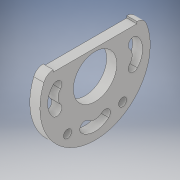
# Autodesk Inventor part: ballast_tengah
Saved by Autodesk Inventor 2019 (Build 230136000, 136)
## iProperties
Created: 2020-07-18
Part Number: ballast_tengah
Material: Generic
Document SubType Name: Modeling
Designer: Agus Prayudi
Density: 1 g/cm^3
Appearance: Default
Author: Agus Prayudi
Autodesk Inventor part; units mm, degrees
ref_plane "YZ Plane" through (0, 0, 0) normal (1, 0, 0) x (0, 1, 0)
ref_plane "XZ Plane" through (0, 0, 0) normal (0, 1, 0) x (-1, 0, 0)
ref_plane "XY Plane" through (0, 0, 0) normal (0, 0, 1) x (1, 0, 0)
sketch "Sketch1" plane through (0, 0, 0) normal (1, 0, 0) x (0, 1, 0)
  arc A0 (13.4228, -41.8269) -> (6.5772, -34.1731) centre (10, -38) ccw
  arc A1 (-13.4228, -41.8269) -> (13.4228, -41.8269) centre (0, -26.8197) ccw
  arc A2 (-6.5772, -34.1731) -> (-13.4228, -41.8269) centre (-10, -38) ccw
  arc A3 (-6.5772, -34.1731) -> (6.5772, -34.1731) centre (0, -26.8197) ccw
  arc A4 (-41.8269, -13.4228) -> (-34.1731, -6.5772) centre (-38, -10) ccw
  arc A5 (-41.8269, 13.4228) -> (-41.8269, -13.4228) centre (-26.8197, 0) ccw
  arc A6 (-34.1731, 6.5772) -> (-41.8269, 13.4228) centre (-38, 10) ccw
  arc A7 (-34.1731, 6.5772) -> (-34.1731, -6.5772) centre (-26.8197, 0) ccw
  arc A8 (-13.4228, 41.8269) -> (-6.5772, 34.1731) centre (-10, 38) ccw
  arc A9 (13.4228, 41.8269) -> (-13.4228, 41.8269) centre (0, 26.8197) ccw
  arc A10 (6.5772, 34.1731) -> (13.4228, 41.8269) centre (10, 38) ccw
  arc A11 (6.5772, 34.1731) -> (-6.5772, 34.1731) centre (0, 26.8197) ccw
  circle A12 centre (0, 0) radius 21.5
  circle A13 centre (-35.3988, 27.25) radius 3.5
  circle A14 centre (-35.3988, -27.25) radius 3.5
  arc A15 (20.2079, 50.6151) -> (20.2079, -50.6151) centre (0, 0) ccw
  line L0 (26.5, -41.328) -> (26.5, 41.328)
  arc A16 (26.5, 41.328) -> (20.2079, 50.6151) centre (16.5, 41.328) ccw
  arc A17 (20.2079, -50.6151) -> (26.5, -41.328) centre (16.5, -41.328) ccw
  point P0 (26.5, -47.6235)
  point P1 (26.5, 47.6235)
  dimension "d4" = 10
  dimension "d5" = 10
  constraints: 32 point on circle, 18 centre point, 4 tangent, 2 end point, 2 point on line
  measures "d4" radius of A16
  measures "d5" radius of A17
extrude "Extrusion1" add sketch "Sketch1" along normal blind 10
sketch "Sketch2" plane through (10, 0, 0) normal (1, 0, 0) x (0, 0, -1)
  line L0 (41.328, 26.5) -> (-41.328, 26.5) projected
  line L1 (0, 24.5) -> (41.328, 24.5)
  line L2 (41.328, 24.5) -> (41.328, 26.5)
  line L3 (0, 24.5) -> (-41.328, 24.5)
  line L4 (-41.328, 24.5) -> (-41.328, 26.5)
  point P0 (0, 0)
  constraints: 8 end point, 1 perpendicular
extrude "Extrusion2" cut sketch "Sketch2" against normal blind 10
sketch "Sketch3" plane through (10, 0, 0) normal (1, 0, 0) x (0, 0, -1)
  circle A0 centre (-27.25, -35.3988) radius 3.5 projected
  circle A1 centre (27.25, -35.3988) radius 3.5 projected
  circle A2 centre (-27.25, -35.3988) radius 4
  circle A3 centre (27.25, -35.3988) radius 4
  point P0 (0, 0)
  dimension "d11" = 8
  dimension "d12" = 8
  constraints: 2 centre point, 2 coincident
  measures "d11" diameter of A2
  measures "d12" diameter of A3
extrude "Extrusion3" cut sketch "Sketch3" against normal blind 10
body "Solid1"
